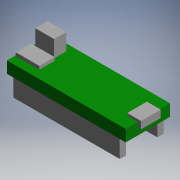
# Autodesk Inventor part: ARDUINO MICRO Simplified
Saved by Autodesk Inventor 2016 (Build 200138000, 138)
## iProperties
Created: 2016-06-09
Part Number: ARDUINO MICRO Simplified
Material: Generic
Document SubType Name: Modeling
Designer: chris
Appearance: Generic
Author: chris
Autodesk Inventor part; units mm, degrees
ref_plane "YZ Plane" through (0, 0, 0) normal (1, 0, 0) x (0, 1, 0)
ref_plane "XZ Plane" through (0, 0, 0) normal (0, 1, 0) x (-1, 0, 0)
ref_plane "XY Plane" through (0, 0, 0) normal (0, 0, 1) x (1, 0, 0)
sketch "Sketch1" plane through (-3.78, -1.3516, -16.62) normal (0, 0, 1) x (1, 0, 0)
  line L0 (0, 0) -> (48.2, 0)
  line L1 (48.2, 0) -> (48.2, 4.7063)
  line L2 (48.2, 4.7063) -> (0, 4.7063)
  line L3 (0, 4.7063) -> (0, 0)
  constraints: 8 end point, 2 parallel, 1 horizontal, 1 perpendicular
extrude "Extrusion1" add sketch "Sketch1" along normal blind 18
sketch "Sketch2" plane through (0, -1.65, -13.93) normal (-1, 0, 0) x (0, 0, 1)
  line L0 (0, 0) -> (5, 0)
  line L1 (5, 0) -> (5, 11.75)
  line L2 (5, 11.75) -> (0, 11.75)
  line L3 (0, 11.75) -> (0, 0)
  constraints: 8 end point, 2 parallel, 1 horizontal, 1 perpendicular
extrude "Extrusion2" add sketch "Sketch2" along normal blind 2.54
sketch "Sketch3" plane through (5.08, -1.65, -13.93) normal (-1, 0, 0) x (0, 0, 1)
  line L0 (0, 0) -> (5, 0)
  line L1 (5, 0) -> (5, 11.75)
  line L2 (5, 11.75) -> (0, 11.75)
  line L3 (0, 11.75) -> (0, 0)
  constraints: 8 end point, 2 parallel, 1 horizontal, 1 perpendicular
extrude "Extrusion3" add sketch "Sketch3" along normal blind 2.54
sketch "Sketch4" plane through (2.54, -1.65, -13.93) normal (-1, 0, 0) x (0, 0, 1)
  line L0 (0, 0) -> (5, 0)
  line L1 (5, 0) -> (5, 11.75)
  line L2 (5, 11.75) -> (0, 11.75)
  line L3 (0, 11.75) -> (0, 0)
  constraints: 8 end point, 2 parallel, 1 horizontal, 1 perpendicular
extrude "Extrusion4" add sketch "Sketch4" along normal blind 2.54
sketch "Sketch5" plane through (-3.5, 1.6, -1.9) normal (1, 0, 0) x (0, 0, -1)
  line L0 (0, 0) -> (6.2, 0)
  line L1 (6.2, 0) -> (6.2, 3.1)
  line L2 (6.2, 3.1) -> (0, 3.1)
  line L3 (0, 3.1) -> (0, 0)
  constraints: 8 end point, 2 parallel, 1 horizontal, 1 perpendicular
extrude "Extrusion5" add sketch "Sketch5" along normal blind 9.6
sketch "Sketch6" plane through (40, 1.3, -3.62) normal (1, 0, 0) x (0, 0, -1)
  line L0 (0, 0) -> (8, 0)
  line L1 (8, 0) -> (8, 2.95)
  line L2 (8, 2.95) -> (0, 2.95)
  line L3 (0, 2.95) -> (0, 0)
  constraints: 8 end point, 2 parallel, 1 horizontal, 1 perpendicular
extrude "Extrusion6" add sketch "Sketch6" along normal blind 5.63
sketch "Sketch7" plane through (41.91, 3.25, -13.97) normal (-1, 0, 0) x (0, 0, -1)
  line L0 (0, 0) -> (2.54, 0)
  line L1 (2.54, 0) -> (2.54, 11.75)
  line L2 (2.54, 11.75) -> (0, 11.75)
  line L3 (0, 11.75) -> (0, 0)
  constraints: 8 end point, 2 parallel, 1 horizontal, 1 perpendicular
extrude "Extrusion7" add sketch "Sketch7" along normal blind 43.18
sketch "Sketch8" plane through (41.91, 3.25, 1.27) normal (-1, 0, 0) x (0, 0, -1)
  line L0 (0, 0) -> (2.54, 0)
  line L1 (2.54, 0) -> (2.54, 11.75)
  line L2 (2.54, 11.75) -> (0, 11.75)
  line L3 (0, 11.75) -> (0, 0)
  constraints: 8 end point, 2 parallel, 1 horizontal, 1 perpendicular
extrude "Extrusion8" add sketch "Sketch8" along normal blind 43.18
body "Solid1"
